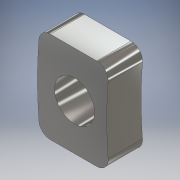
# Autodesk Inventor part: reverse gear link block
Saved by Autodesk Inventor 2017 (Build 210142000, 142)
## iProperties
Created: 2018-11-03
Part Number: reverse gear link block
Material: Generic
Document SubType Name: Modeling
Designer: User
Density: 1 g/cm^3
Appearance: Default
Author: User
Autodesk Inventor part; units mm, degrees
ref_plane "YZ Plane" through (0, 0, 0) normal (1, 0, 0) x (0, 1, 0)
ref_plane "XZ Plane" through (0, 0, 0) normal (0, 1, 0) x (-1, 0, 0)
ref_plane "XY Plane" through (0, 0, 0) normal (0, 0, 1) x (1, 0, 0)
sketch "Sketch1" plane through (0, 0, 0) normal (0, 1, 0) x (-1, 0, 0)
  arc A0 (0, -35.5) -> (0, 35.5) centre (0, 0) ccw construction
  arc A1 (-2.5809, -40.3369) -> (-17.4082, 36.0494) centre (1.0497, 0) ccw construction
  arc A2 (39.0973, -13.8791) -> (40.8076, 7.7173) centre (1.0497, 0) ccw construction
  line L0 (41.5497, -0.0049) -> (41.3517, -4) construction
  line L1 (41.5497, -0.0049) -> (41.3527, 3.9902) construction
  arc A3 (41.3517, -4) -> (41.3527, 3.9902) centre (1.0497, 0) ccw
  line L2 (35.5, 0) -> (35.5, -4) construction
  line L3 (35.5, 0) -> (35.5, 4) construction
  arc A4 (35.2739, -4) -> (35.275, 3.9902) centre (0, 0) ccw construction
  arc A5 (35.2739, -4) -> (35.275, 3.9902) centre (0, 0) ccw
  line L4 (41.3527, 3.9902) -> (35.275, 3.9902)
  line L5 (41.3517, -4) -> (35.2739, -4)
  dimension "d7" = 0
  dimension "d8" = 40.5
  dimension "d9" = 35.5
  dimension "d14" = 4
  dimension "d15" = 4
  dimension "d18" = 4
  dimension "d19" = 4
  constraints: 24 point on circle, 12 end point, 6 centre point, 2 tangent, 2 vertical, 1 concentric, 1 horizontal, 1 parallel
  measures "d7" vertical distance of A1.centre A0.centre
  measures "d8" radius of A1
  measures "d9" radius of A0
  measures "d14" distance of L0.start L0.end
  measures "d15" distance of L0.start L1.end
  measures "d18" distance of L2.start L2.end
  measures "d19" distance of L2.start L3.end
extrude "Extrusion1" add sketch "Sketch1" along normal blind 3
sketch "Sketch2" plane through (0, 3, 0) normal (0, 1, 0) x (1, 0, 0)
  arc A0 (-41.3517, 4) -> (-41.3527, -3.9902) centre (-1.0497, 0) ccw projected
  line L0 (-41.3527, -3.9902) -> (-35.275, -3.9902) projected
  arc A1 (-35.2739, 4) -> (-35.275, -3.9902) centre (0, 0) ccw projected
  line L1 (-35.2739, 4) -> (-41.3517, 4) projected
  circle A2 centre (-38.3128, 0) radius 1.75
  point P0 (0, 0)
  dimension "d22" = 3.5
  constraints: 1 centre point
  measures "d22" diameter of A2
extrude "Extrusion2" cut sketch "Sketch2" along normal through all both and the other way through all contours A2
fillet "Fillet1" radius 1 4 edges at (-41.3527, 1.5, 3.9902) (-41.3517, 1.5, -4) (-35.2739, 1.5, -4) (-35.275, 1.5, 3.9902)
body "Solid1"
